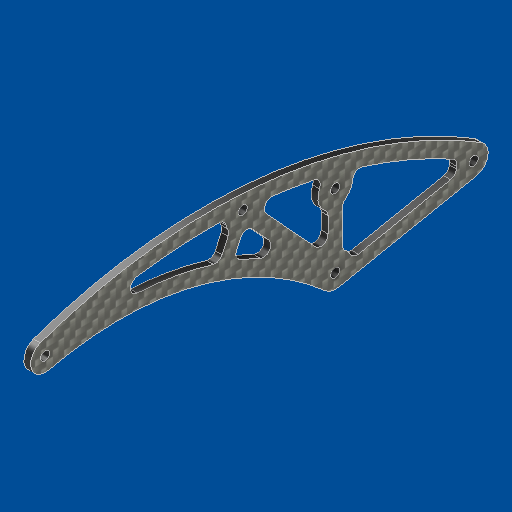
# Autodesk Inventor part: upperArmHanger
Saved by Autodesk Inventor 2023 (Build 270158030, 158C)
## iProperties
Created: 2023-03-03
Part Number: upperArmHanger
Material: CFRP
Document SubType Name: Modeling
Designer: kumpu
Density: 1.43 g/cm^3
Appearance: Glossy - Black
Author: kumpu
Autodesk Inventor part; units mm, degrees
ref_plane "YZ Plane" through (0, 0, 0) normal (1, 0, 0) x (0, 1, 0)
ref_plane "XZ Plane" through (0, 0, 0) normal (0, 1, 0) x (-1, 0, 0)
ref_plane "XY Plane" through (0, 0, 0) normal (0, 0, 1) x (1, 0, 0)
sketch "Sketch1" plane through (0, 0, 0) normal (1, 0, 0) x (0, 1, 0)
  circle A0 centre (0, 0) radius 13.462
  circle A1 centre (22.0533, -125.0706) radius 2
  line L0 (22.0533, -125.0706) -> (0, 0) construction
  circle A2 centre (0, 0) radius 35 construction
  circle A3 centre (10, -64.4908) radius 2 projected
  circle A4 centre (42, -64.4908) radius 2 projected
  circle A5 centre (54, -23.9908) radius 2 projected
  circle A6 centre (42, 62.5092) radius 2 projected
  line L1 (42, -64.4908) -> (10, -64.4908) construction
  line L2 (15.8254, -126.3097) -> (3.7721, -65.7299)
  arc A7 (15.8254, -126.3097) -> (27.4672, -128.3891) centre (22.0533, -125.0706) ccw
  arc A8 (47.9907, 64.615) -> (35.8225, 61.0392) centre (42, 62.5092) ccw
  circle A9 centre (54, -23.9908) radius 6.35 construction
  arc A10 (5.2567, -60.269) -> (3.7721, -65.7299) centre (10, -64.4908) ccw
  arc A11 (5.2567, -60.269) -> (35.8225, 61.0392) centre (-95.8375, 29.7084) ccw
  arc A12 (27.4672, -128.3891) -> (47.9907, 64.615) centre (-165.1613, -10.3123) ccw
  line L3 (10, -64.4908) -> (42, 62.5092) construction
  line L4 (42, 62.5092) -> (54, -23.9908) construction
  line L5 (54, -23.9908) -> (10, -64.4908) construction
  line L6 (42, -64.4908) -> (54, -23.9908) construction
  line L7 (22.0533, -125.0706) -> (10, -64.4908) construction
  line L8 (22.0533, -125.0706) -> (42, -64.4908) construction
  line L9 (54, -23.9908) -> (0, 0) construction
  arc A13 (25.9223, -118.5059) -> (45.8555, -71.0634) centre (-165.1613, -10.3123) ccw
  arc A14 (35.073, -67.6658) -> (45.8555, -71.0634) centre (42, -64.4908) ccw
  arc A15 (11.487, -71.9643) -> (16.927, -67.6658) centre (10, -64.4908) ccw
  arc A16 (25.9223, -118.5059) -> (20.5663, -117.5971) centre (22.0533, -125.0706) ccw
  line L10 (20.5663, -117.5971) -> (11.487, -71.9643)
  line L11 (16.927, -67.6658) -> (35.073, -67.6658)
  line L12 (35.073, -61.3158) -> (18.1375, -61.3158)
  arc A17 (48.5796, -60.6472) -> (35.073, -61.3158) centre (42, -64.4908) ccw
  arc A18 (48.5796, -60.6472) -> (53.3935, -31.5866) centre (-165.1613, -10.3123) ccw
  arc A19 (51.0536, -31.0181) -> (53.3935, -31.5866) centre (54, -23.9908) ccw
  line L13 (18.1375, -61.3158) -> (51.0536, -31.0181)
  line L14 (21.7098, -49.3972) -> (46.7531, -26.346)
  line L15 (46.3805, -24.0799) -> (36.8936, -19.8651)
  line L16 (48.9587, -18.2768) -> (38.9882, -13.8472)
  arc A20 (21.7098, -49.3972) -> (36.8936, -19.8651) centre (-95.8375, 29.7084) ccw
  arc A21 (54.3426, -16.3785) -> (51.9599, 22.5079) centre (-165.1613, -10.3123) ccw
  arc A22 (51.9599, 22.5079) -> (45.65, 22.2016) centre (48.8206, 22.0334) ccw
  arc A23 (38.9882, -13.8472) -> (45.65, 22.2016) centre (-95.8375, 29.7084) ccw
  arc A24 (22.0533, -125.0706) -> (42, 62.5092) centre (-165.1613, -10.3123) ccw construction
  circle A25 centre (10, -64.4908) radius 3.175 construction
  circle A26 centre (54, -23.9908) radius 3.175 construction
  arc A27 (46.3805, -24.0799) -> (46.7531, -26.346) centre (54, -23.9908) ccw
  arc A28 (54.3426, -16.3785) -> (48.9587, -18.2768) centre (54, -23.9908) ccw
  dimension "d0" = 26.924
  dimension "d1" = 4
  dimension "d2" = 70
  dimension "d3" = 127
  dimension "d4" = 80
  dimension "d5" = 6.35
  dimension "d6" = 6.35
  dimension "d7" = 7.62
  dimension "d8" = 3.175
  constraints: 40 point on circle, 34 end point, 25 centre point, 18 concentric, 17 tangent, 14 equal radius, 4 parallel, 3 coincident, 2 horizontal, 1 collinear
  measures "d0" diameter of A0
  measures "d1" diameter of A1
  measures "d2" diameter of A2
  measures "d3" distance of L0.start L0.end
  measures "d4" angle of L0 L1
  measures "d5" radius of A8
  measures "d6" diameter of A25
  measures "d7" radius of A17
  measures "d8" radius of A22
extrude "Extrusion1" add sketch "Sketch1" along normal blind 3 contours L2 A10 A11 A8 A12 A7
fillet "Fillet1" radius 3.175 18 edges at (1.5, 20.5663, -117.5971) (1.5, 11.487, -71.9643) (1.5, 25.9223, -118.5059) (1.5, 45.8555, -71.0634) (1.5, 35.073, -67.6658) (1.5, 16.927, -67.6658) (1.5, 48.5796, -60.6472) (1.5, 35.073, -61.3158) (1.5, 53.3935, -31.5866) (1.5, 51.0536, -31.0181) (1.5, 18.1375, -61.3158) (1.5, 46.3805, -24.0799) (1.5, 46.7531, -26.346) (1.5, 36.8936, -19.8651) (1.5, 21.7098, -49.3972) (1.5, 54.3426, -16.3785) (1.5, 48.9587, -18.2768) (1.5, 38.9882, -13.8472)
body "Solid1"
